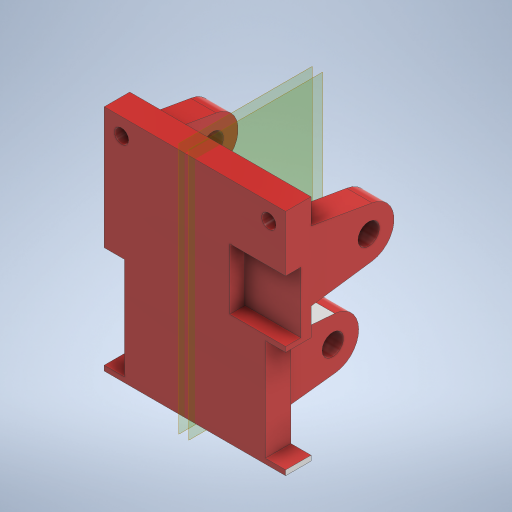
# Autodesk Inventor part: Качель камеры
Saved by Autodesk Inventor 2023 (Build 270158000, 158)
## iProperties
Created: 2024-02-27
Part Number: Качель камеры
Material: Типовые
Document SubType Name: Modeling
Designer: liza
Density: 1 g/cm^3
Appearance: По умолчанию
Author: liza
Autodesk Inventor part; units mm, degrees
ref_plane "YZ Plane" through (0, 0, 0) normal (1, 0, 0) x (0, 1, 0)
ref_plane "XZ Plane" through (0, 0, 0) normal (0, 1, 0) x (-1, 0, 0)
ref_plane "XY Plane" through (0, 0, 0) normal (0, 0, 1) x (1, 0, 0)
sketch "Эскиз1" plane through (0, 0, 0) normal (0, 0, 1) x (1, 0, 0)
  line L0 (0, 0) -> (35.65, 0)
  line L1 (35.65, 0) -> (35.65, -45)
  line L2 (35.65, -45) -> (0, -45)
  line L3 (0, -45) -> (0, 0)
  dimension "d0" = 35.65
  dimension "d1" = 45
  constraints: 8 end point, 2 parallel, 1 horizontal, 1 perpendicular
  measures "d0" distance of L0.start L0.end
  measures "d1" distance of L0.end L1.end
extrude "Выдавливание1" add sketch "Эскиз1" along normal blind 5
sketch "Эскиз5" plane through (0, -45, 0) normal (-1, 0, 0) x (0, 0, 1)
  line L0 (0, 0) -> (0, 45) projected
  line L1 (0, 26.3892) -> (-12, 28.047)
  circle A0 centre (-11.3157, 33) radius 5
  circle A1 centre (-11.3157, 33) radius 2.1
  line L2 (0, 45) -> (5, 45) projected
  line L3 (-12, 37.953) -> (0, 40.0416)
  point P0 (0, 38.3892)
  point P1 (-10.5919, 37.9473)
  point P2 (-11.2301, 37.9993)
  point P3 (0, 41.0557)
  dimension "d4" = 4.2
  dimension "d5" = 10
  dimension "d8" = 12
  dimension "d9" = 12
  dimension "d10" = 12
  dimension "d18" = 12
  constraints: 4 end point, 4 point on circle, 4 point on line, 2 centre point, 1 coincident, 1 tangent
  measures "d4" diameter of A1
  measures "d5" diameter of A0
  measures "d8" horizontal distance of L1.start L1.end
  measures "d9" distance from line of A1.centre L2
  measures "d10" distance of L1.start point (0, 38.389)
  measures "d18" horizontal distance of L3.end L3.start
extrude "Выдавливание2" add sketch "Эскиз5" against normal blind 5
ref_plane "РабПлоскость1" through (17.825, -45, 5) normal (-1, 0, 0) x (0, 0, 1)
mirror "Зеркальное отражение1" about plane through (17.825, -45, 5) normal (-1, 0, 0) of "Выдавливание2"
sketch "Эскиз7" plane through (0, 0, 0) normal (0, 0, -1) x (-1, 0, 0)
  circle A0 centre (-32.35, -3.3) radius 1.4 projected
  circle A1 centre (-3.39, -3.3) radius 1.4 projected
  line L0 (-3.9799, -24) -> (1.0201, -24)
  line L1 (1.0201, -24) -> (1.0201, -44)
  line L2 (1.0201, -44) -> (-3.9799, -44)
  line L3 (-3.9799, -44) -> (-3.9799, -24)
  line L4 (0, -45) -> (-35.65, -45) construction
  line L5 (-17.825, -45) -> (-17.825, 0) construction
  line L6 (-35.65, 0) -> (0, 0) construction
  line L7 (-31.6701, -24) -> (-36.6701, -24)
  line L8 (-36.6701, -24) -> (-36.6701, -44)
  line L9 (-36.6701, -44) -> (-31.6701, -44)
  line L10 (-31.6701, -44) -> (-31.6701, -24)
  line L11 (0, 0) -> (0, -45) construction
  point P0 (0, -18.6108)
  dimension "d14" = 1
  dimension "d15" = 20
  dimension "d24" = 5
  constraints: 18 end point, 4 symmetric about line, 2 midpoint, 2 parallel, 1 horizontal, 1 perpendicular
  measures "d14" distance between parallel lines of L4 L2
  measures "d15" distance of L2.end L0.start
  measures "d24" distance of L0.start L0.end
extrude "Выдавливание3" cut sketch "Эскиз7" against normal through all
sketch "Эскиз9" plane through (0, 0, 5) normal (0, 0, 1) x (1, 0, 0)
  line L0 (35.65, -45) -> (35.65, 0) projected
  line L1 (35.65, -11) -> (24.65, -11)
  line L2 (24.65, -11) -> (24.65, -23)
  line L3 (24.65, -23) -> (35.65, -23)
  line L4 (35.65, -23) -> (35.65, -11)
  point P0 (0, 0)
  dimension "d19" = 11
  dimension "d20" = 12
  dimension "d21" = 11
  constraints: 8 end point, 2 parallel, 1 horizontal, 1 perpendicular, 1 point on line
  measures "d19" distance of L1.start L0.end
  measures "d20" distance of L1.end L2.end
  measures "d21" distance of L2.end L3.end
extrude "Выдавливание4" cut sketch "Эскиз9" against normal blind 3
ref_plane "РабПлоскость2" through (15.825, -45, 5) normal (-1, 0, 0) x (0, 0, 1)
sketch "Эскиз10" plane through (15.825, -45, 5) normal (-1, 0, 0) x (0, 0, 1)
  circle A0 centre (-20.0926, 6.8885) radius 5.1
  circle A1 centre (-20.0926, 6.8885) radius 2.1
  line L0 (-20.6814, 1.8226) -> (-5, 0)
  line L1 (-5, 11.6783) -> (-5, 0)
  line L2 (-20.4955, 11.9725) -> (-5, 13.2004)
  line L3 (-5, 1) -> (-5, 21) projected
  point P0 (-5, 45)
  point P1 (-20.9797, 11.9107)
  point P2 (-22.1404, 2.2176)
  point P3 (-20.6271, 11.9604)
  dimension "d28" = 4.2
  dimension "d29" = 10.2
  constraints: 6 end point, 5 point on circle, 2 centre point, 2 tangent, 1 coincident, 1 point on line, 1 vertical
  measures "d28" diameter of A1
  measures "d29" diameter of A0
extrude "Выдавливание5" add sketch "Эскиз10" along normal blind 5
mirror "Зеркальное отражение2" about plane through (17.825, -45, 5) normal (-1, 0, 0) of "Выдавливание5"
